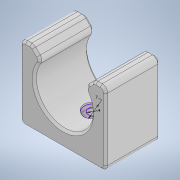
# Autodesk Inventor part: conduit_holder
Saved by Autodesk Inventor 2020.3 (Build 243373000, 373)
## iProperties
Created: 2020-06-22
Part Number: conduit_holder
Material: Generic
Document SubType Name: Modeling
Designer: OskarJohansson
Density: 1 g/cm^3
Appearance: Default
Author: OskarJohansson
## iProperties of the stored document _3DPrint.ipt
Created: 2020-06-22
Part Number: _3DPrint
Material: Generic
Document SubType Name: Modeling
Designer: OskarJohansson
Density: 1 g/cm^3
Appearance: Default
Author: OskarJohansson
Autodesk Inventor part; units mm, degrees
ref_plane "YZ Plane" through (0, 0, 0) normal (1, 0, 0) x (0, 1, 0)
ref_plane "XZ Plane" through (0, 0, 0) normal (0, 1, 0) x (-1, 0, 0)
ref_plane "XY Plane" through (0, 0, 0) normal (0, 0, 1) x (1, 0, 0)
sketch "Sketch1" plane through (0, 0, 0) normal (0, 0, 1) x (1, 0, 0)
  arc A0 (0, 0) -> (7.8262, 17.5) centre (0, 10.5) ccw
  line L0 (0, 26.4) -> (0, -11.4) projected
  line L1 (-48.3956, 0) -> (48.6087, 0) projected
  line L2 (7.8262, 17.5) -> (11.3262, 21)
  line L3 (11.3262, 21) -> (15.75, 21)
  line L4 (15.75, 21) -> (15.75, -6)
  line L5 (15.75, -6) -> (0, -6)
  arc A1 (-7.8262, 17.5) -> (0, 0) centre (0, 10.5) ccw
  line L6 (48.3956, 0) -> (-48.6087, 0)
  line L7 (-7.8262, 17.5) -> (-11.3262, 21)
  line L8 (-11.3262, 21) -> (-15.75, 21)
  line L9 (-15.75, 21) -> (-15.75, -6)
  line L10 (-15.75, -6) -> (0, -6)
  dimension "d0" = 10.5
  dimension "d1" = 17.5
  dimension "d2" = 45
  dimension "d3" = 15.75
  dimension "d4" = 21
  dimension "d5" = 6
  constraints: 18 end point, 6 point on circle, 6 symmetric about line, 3 point on line, 2 centre point, 2 horizontal, 1 perpendicular, 1 tangent, 1 other
  measures "d0" radius of A0
  measures "d1" distance from line of L1 L2.start
  measures "d2" angle of L2 L3
  measures "d3" distance between parallel lines of L0 L4
  measures "d4" distance between parallel lines of L1 L3
  measures "d5" distance between parallel lines of L5 L1
extrude "Extrusion1" add sketch "Sketch1" along normal blind 20
sketch "Sketch2" plane through (0, 0, 0) normal (0, 1, 0) x (-1, 0, 0)
  circle A0 centre (0, 8.6607) radius 2
  circle A1 centre (0, 8.6607) radius 3.5
  point P0 (0, 0)
  dimension "d8" = 7
  dimension "d9" = 4
  constraints: 2 centre point, 1 coincident
  measures "d8" diameter of A1
  measures "d9" diameter of A0
extrude "Extrusion2" cut sketch "Sketch2" along normal through all both and the other way through all contours A0
extrude "Extrusion3" cut sketch "Sketch2" along normal blind 10 and the other way blind 3 contours A0 | A1
chamfer "Chamfer1" distance 1.5 angle 45 1 edges at (3.5, -3, 8.6607)
fillet "Fillet1" radius 2 8 edges at (-15.75, -6, 10) (15.75, -6, 10) (7.8262, 17.5, 10) (11.3262, 21, 10) (15.75, 21, 10) (-7.8262, 17.5, 10) (-11.3262, 21, 10) (-15.75, 21, 10)
chamfer "Chamfer2" distance 0.8 angle 45 32 edges at (-15.75, 7.5, 20) (-15.1642, -5.4142, 20) (0, -6, 20) (15.1642, -5.4142, 20) (15.75, 7.5, 20) (15.1642, 20.4142, 20) (12.9523, 21, 20) (11.3893, 20.8478, 20) (9.9007, 19.5745, 20) (8.486, 17.5284, 20) (0, 0, 20) (-8.486, 17.5284, 20) (-9.9007, 19.5745, 20) (-11.3893, 20.8478, 20) (-12.9523, 21, 20) (-15.1642, 20.4142, 20) (15.75, 7.5, 0) (15.1642, 20.4142, 0) (12.9523, 21, 0) (11.3893, 20.8478, 0) (9.9007, 19.5745, 0) (8.486, 17.5284, 0) (0, 0, 0) (-8.486, 17.5284, 0) (-9.9007, 19.5745, 0) (-11.3893, 20.8478, 0) (-12.9523, 21, 0) (-15.1642, 20.4142, 0) (-15.75, 7.5, 0) (-15.1642, -5.4142, 0) (0, -6, 0) (15.1642, -5.4142, 0)
equation "\"d1\" = 1.66667 * d0"
equation "\"d3\" = 1.5 * d0"
equation "\"d4\" = 2 * d0"
equation "\"D_Screw\" = 4"
equation "\"D_Screwhead\" = 6"
body "Solid1"
